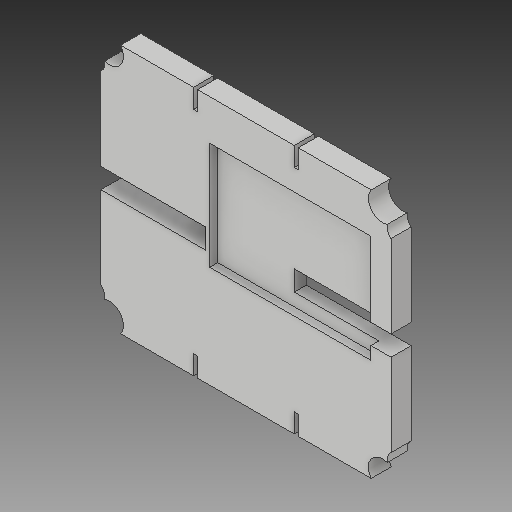
# Autodesk Inventor part: Каркас
Saved by Autodesk Inventor 2019 (Build 230136000, 136)
## iProperties
Created: 2020-05-20
Part Number: Каркас
Material: Типовые
Document SubType Name: Modeling
Designer: Surflay
Density: 1 g/cm^3
Appearance: По умолчанию
Author: Surflay
Autodesk Inventor part; units mm, degrees
ref_plane "YZ Plane" through (0, 0, 0) normal (1, 0, 0) x (0, 1, 0)
ref_plane "XZ Plane" through (0, 0, 0) normal (0, 1, 0) x (-1, 0, 0)
ref_plane "XY Plane" through (0, 0, 0) normal (0, 0, 1) x (1, 0, 0)
sketch "Эскиз1" plane through (0, 0, 0) normal (0, 0, 1) x (1, 0, 0)
  line L0 (174.3111, 41.624) -> (226.3111, 41.624) projected
  line L1 (134.3111, 31.624) -> (82.3111, 31.624) projected
  line L2 (174.3111, 41.624) -> (174.3111, 31.624) projected
  line L3 (149.3111, 46.624) -> (159.3111, 46.624) projected
  line L4 (149.3111, 46.624) -> (149.3111, 86.624) projected
  line L5 (149.3111, 86.624) -> (159.3111, 86.624) projected
  line L6 (159.3111, 86.624) -> (159.3111, 46.624) projected
  line L7 (134.3111, 31.624) -> (134.3111, 41.624) projected
  line L8 (226.3111, 31.624) -> (174.3111, 31.624) projected
  line L9 (82.3111, 41.624) -> (134.3111, 41.624) projected
  line L10 (226.3111, 41.624) -> (226.3111, 82.624) projected
  arc A0 (216.499, 98.624) -> (224.45, 87.7942) centre (222.0611, 94.374) ccw projected
  line L11 (216.499, 98.624) -> (180.3111, 98.624) projected
  line L12 (180.3111, 98.624) -> (180.3111, 89.124) projected
  line L13 (180.3111, 89.124) -> (178.3111, 89.124) projected
  line L14 (178.3111, 89.124) -> (178.3111, 98.624) projected
  line L15 (178.3111, 98.624) -> (130.3111, 98.624) projected
  line L16 (130.3111, 98.624) -> (130.3111, 89.124) projected
  line L17 (130.3111, 89.124) -> (128.3111, 89.124) projected
  line L18 (128.3111, 89.124) -> (128.3111, 98.624) projected
  line L19 (128.3111, 98.624) -> (92.1233, 98.624) projected
  arc A1 (84.1722, 87.7942) -> (92.1233, 98.624) centre (86.5611, 94.374) ccw projected
  line L20 (82.3111, -9.376) -> (82.3111, 31.624) projected
  arc A2 (92.1233, -25.376) -> (84.1722, -14.5463) centre (86.5611, -21.126) ccw projected
  line L21 (128.3111, -25.376) -> (92.1233, -25.376) projected
  line L22 (128.3111, -25.376) -> (128.3111, -15.876) projected
  line L23 (128.3111, -15.876) -> (130.3111, -15.876) projected
  line L24 (130.3111, -15.876) -> (130.3111, -25.376) projected
  line L25 (178.3111, -25.376) -> (130.3111, -25.376) projected
  line L26 (178.3111, -25.376) -> (178.3111, -15.876) projected
  line L27 (178.3111, -15.876) -> (180.3111, -15.876) projected
  line L28 (180.3111, -15.876) -> (180.3111, -25.376) projected
  line L29 (216.499, -25.376) -> (180.3111, -25.376) projected
  arc A3 (224.45, -14.5463) -> (216.499, -25.376) centre (222.0611, -21.126) ccw projected
  line L30 (159.3111, 26.624) -> (149.3111, 26.624) projected
  line L31 (159.3111, 26.624) -> (159.3111, -13.376) projected
  line L32 (159.3111, -13.376) -> (149.3111, -13.376) projected
  line L33 (149.3111, -13.376) -> (149.3111, 26.624) projected
  arc A4 (224.45, 87.7942) -> (226.3111, 82.624) centre (229.3111, 86.624) ccw projected
  arc A5 (84.1722, -14.5463) -> (82.3111, -9.376) centre (79.3111, -13.376) ccw projected
  arc A6 (82.3111, 82.624) -> (84.1722, 87.7942) centre (79.3111, 86.624) ccw projected
  arc A7 (226.3111, -9.376) -> (224.45, -14.5463) centre (229.3111, -13.376) ccw projected
  line L34 (226.3111, -9.376) -> (226.3111, 31.624) projected
  line L35 (82.3111, 41.624) -> (82.3111, 82.624) projected
  point P0 (0, 0)
  point P1 (179.3111, -15.876)
  point P2 (129.3111, -15.876)
  point P3 (70.835, 120.6534)
  point P4 (129.3111, 89.124)
  point P5 (179.3111, 89.124)
  point P6 (242.2845, 49.4059)
  point P7 (79.3111, -13.376)
  point P8 (229.3111, -13.376)
  constraints: 4 midpoint
extrude "Выдавливание1" add sketch "Эскиз1" along normal blind 10 contours L2 L8 L34 A7 A3 L29 L28 L27 L26 L25 L24 L23 L22 L21 A2 A5 L20 L1 L7 L9 L35 A6 A1 L19 L18 L17 L16 L15 L14 L13 L12 L11 A0 A4 L10 L0 | L4 L5 L6 L3 | L31 L32 L33 L30
sketch "Эскиз2" plane through (0, 0, 10) normal (0, 0, 1) x (1, 0, 0)
  line L0 (216.3111, 25.284) -> (136.3111, 25.284)
  line L1 (136.3111, 25.284) -> (136.3111, 78.624)
  line L2 (136.3111, 78.624) -> (216.3111, 78.624)
  line L3 (216.3111, 78.624) -> (216.3111, 25.284)
  line L4 (226.3111, 41.624) -> (226.3111, 82.624) projected
  line L5 (216.499, 98.624) -> (180.3111, 98.624) projected
  point P0 (0, 0)
  point P1 (231.3111, -8.7934)
  point P2 (231.3111, 82.0414)
  point P3 (226.3111, 82.624)
  dimension "d14" = 80
  dimension "d15" = 53.34
  dimension "d58" = 20
  dimension "d59" = 10
  constraints: 8 end point, 2 parallel, 1 horizontal, 1 perpendicular, 1 other
  measures "d14" distance of L0.start L0.end
  measures "d15" distance of L0.end L1.end
  measures "d58" distance between parallel lines of L5 L2
extrude "Выдавливание2" cut sketch "Эскиз2" against normal blind 4
